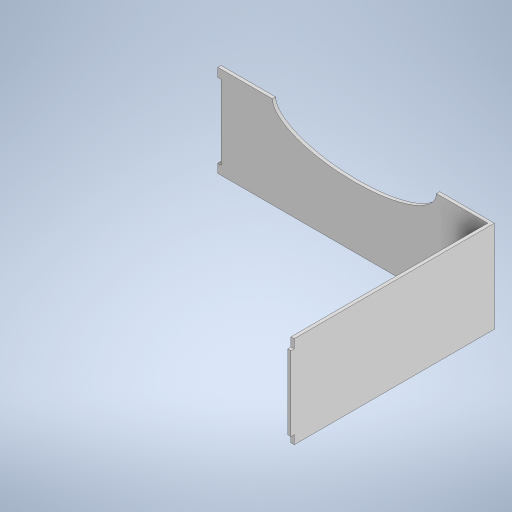
# Autodesk Inventor part: передняя стенка
Saved by Autodesk Inventor 2024.2 (Build 282272000, 272)
## iProperties
Created: 2025-11-20
Part Number: передняя стенка
Material: Типовые
Document SubType Name: Modeling
Designer: Zakhar
Density: 1 g/cm^3
Appearance: По умолчанию
Author: Zakhar
Autodesk Inventor part; units mm, degrees
ref_plane "YZ Plane" through (0, 0, 0) normal (1, 0, 0) x (0, 1, 0)
ref_plane "XZ Plane" through (0, 0, 0) normal (0, 1, 0) x (-1, 0, 0)
ref_plane "XY Plane" through (0, 0, 0) normal (0, 0, 1) x (1, 0, 0)
sketch "Эскиз1" plane through (0, 0, 0) normal (1, 0, 0) x (0, 1, 0)
  line L0 (84, 90) -> (0, 90)
  line L1 (0, 90) -> (0, -90)
  line L2 (0, -90) -> (84, -90)
  line L3 (84, -90) -> (84, 90)
  line L4 (76, 90) -> (8, 90)
  line L5 (8, 90) -> (8, 93)
  line L6 (8, 93) -> (76, 93)
  line L7 (76, 93) -> (76, 90)
  line L8 (76, -90) -> (8, -90)
  line L9 (8, -90) -> (8, -93)
  line L10 (8, -93) -> (76, -93)
  line L11 (76, -93) -> (76, -90)
  point P0 (0, 0)
  point P1 (76, 91.5)
  point P2 (8, 91.5)
  point P3 (8, -90)
  dimension "d0" = 180
  dimension "d1" = 84
  dimension "d2" = 90
  dimension "d3" = 0
  dimension "d4" = 3
  dimension "d5" = 8
  dimension "d6" = 8
  dimension "d7" = 3
  constraints: 24 end point, 6 parallel, 4 point on line, 3 horizontal, 3 perpendicular, 2 midpoint
  measures "d0" distance of L0.end L1.end
  measures "d1" distance of L0.start L0.end
  measures "d2" distance from line of point (0, 0) L2
  measures "d3" distance from line of L1 point (0, 0)
  measures "d4" distance of L6.end L4.start
  measures "d5" horizontal distance of L0.start point (76, 91.5)
  measures "d6" horizontal distance of L0.end point (8, 91.5)
  measures "d7" distance between parallel lines of L2 L10
extrude "Выдавливание1" add sketch "Эскиз1" along normal blind 3
sketch "Эскиз2" plane through (0, 76, -90) normal (0, 0, -1) x (-1, 0, 0)
  line L0 (247, 8) -> (247, -76)
  line L1 (247, -76) -> (-3, -76)
  line L2 (-3, -76) -> (-3, 8)
  line L3 (0, -76) -> (-3, -76) projected
  line L4 (0, 0) -> (-3, 0) projected
  line L5 (0, -76) -> (0, -68) projected
  line L6 (-3, 0) -> (0, 0)
  line L7 (0, 0) -> (0, -68)
  line L8 (0, -68) -> (-3, -68)
  line L9 (-3, -68) -> (-3, 0)
  ellipse E0 centre (122, 8) end of major axis (197, 8) minor radius 28.3094 (47, 8) -> (197, 8) ccw
  line L10 (-3, 8) -> (47, 8)
  line L11 (197, 8) -> (247, 8)
  line L12 (247, 0) -> (244, 0)
  line L13 (244, 0) -> (244, -68)
  line L14 (244, -68) -> (247, -68)
  line L15 (247, -68) -> (247, 0)
  point P0 (245.5, -68)
  dimension "d13" = 75
  dimension "d10" = 250
  dimension "d14" = 125
  dimension "d15" = 84
  dimension "d16" = 150
  dimension "d17" = 84
  dimension "d18" = 3
  dimension "d19" = 8
  constraints: 26 end point, 7 parallel, 4 horizontal, 4 perpendicular, 1 collinear, 1 midpoint, 1 point on line, 4 other
  measures "d10" distance of L0.end L1.end
  measures "d14" distance of L0.start point (122, 8)
  measures "d15" distance between parallel lines of L1 L11
  measures "d16" distance of L10.end L11.start
  measures "d17" distance from line of L1 point (122, 8)
  measures "d18" distance of L12.start L12.end
  measures "d19" vertical distance of point (245.5, -68) L0.end
extrude "Выдавливание2" add sketch "Эскиз2" along normal blind 3 contours L0 L12 L13 L14 L1 L5 L7 L4 L2 L10 E0 L11 | L1 L2 L8 L5
equation "\"d2\" = 0.5 * d0"
